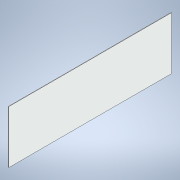
# Autodesk Inventor part: acrilicoMovel1
Saved by Autodesk Inventor 2022 (Build 260153000, 153)
## iProperties
Created: 2022-08-29
Part Number: acrilicoMovel1
Material: Generic
Document SubType Name: Modeling
Designer: cvss2
Density: 1 g/cm^3
Appearance: Default
Author: cvss2
Autodesk Inventor part; units mm, degrees
ref_plane "YZ Plane" through (0, 0, 0) normal (1, 0, 0) x (0, 1, 0)
ref_plane "XZ Plane" through (0, 0, 0) normal (0, 1, 0) x (-1, 0, 0)
ref_plane "XY Plane" through (0, 0, 0) normal (0, 0, 1) x (1, 0, 0)
sketch "Sketch1" plane through (0, 0, 0) normal (1, 0, 0) x (0, 1, 0)
  line L0 (0, 0) -> (-470, 0)
  line L1 (-470, 0) -> (-470, 1118)
  line L2 (-470, 1118) -> (0, 1118)
  line L3 (0, 1118) -> (0, 0)
  dimension "d0" = 470
  dimension "d1" = 1118
  constraints: 8 end point, 2 parallel, 1 horizontal, 1 perpendicular
  measures "d0" distance of L1.end L2.end
  measures "d1" distance of L0.end L1.end
extrude "Extrusion1" add sketch "Sketch1" against normal blind 3
equation "\"d0\" = portaLargura"
equation "\"portaLarguraOld\" = 363"
equation "\"portaAltura\" = 1138"
equation "\"portaLargura\" = 470"
body "Solid1"
